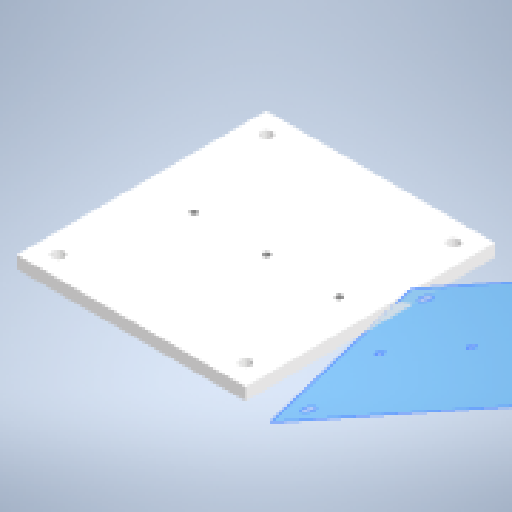
# Autodesk Inventor part: Deska izolovaná
Saved by Autodesk Inventor 2023 (Build 270158000, 158)
## iProperties
Created: 2023-03-26
Part Number: Deska izolovaná
Material: PC/ABS Plastic
Document SubType Name: Modeling
Designer: lukyv
Density: 0.357273 g/cm^3
Appearance: Smooth - White
Author: lukyv
Autodesk Inventor part; units mm, degrees
ref_plane "YZ Plane" through (0, 0, 0) normal (1, 0, 0) x (0, 1, 0)
ref_plane "XZ Plane" through (0, 0, 0) normal (0, 1, 0) x (-1, 0, 0)
ref_plane "XY Plane" through (0, 0, 0) normal (0, 0, 1) x (1, 0, 0)
sketch "Sketch1" plane through (0, 0, 0) normal (0, 1, 0) x (-1, 0, 0)
  line L0 (0, 0) -> (110, 0)
  line L1 (110, 0) -> (110, -110)
  line L2 (110, -110) -> (0, -110)
  line L3 (0, -110) -> (0, 0)
  circle A0 centre (5, -5) radius 2.75
  line L4 (55, 0) -> (55, -110) construction
  line L5 (0, -55) -> (110, -55) construction
  circle A1 centre (5, -105) radius 2.75
  circle A2 centre (105, -5) radius 2.75
  circle A3 centre (105, -105) radius 2.75
  dimension "d0" = 110
  dimension "d1" = 110
  dimension "d2" = 5.5
  dimension "d5" = 100
  dimension "d8" = 100
  dimension "d11" = 5
  dimension "d12" = 5
  constraints: 12 end point, 4 centre point, 4 midpoint, 2 horizontal, 2 parallel, 1 perpendicular, 1 vertical, 6 other
  measures "d0" distance of L1.end L2.end
  measures "d1" distance of L0.end L1.end
  measures "d2" diameter of A0
  measures "d5" distance of A0.centre A1.centre
  measures "d8" distance of A0.centre A2.centre
  measures "d11" distance from line of L0 A0.centre
  measures "d12" distance from line of L3 A0.centre
extrude "Extrusion1" add sketch "Sketch1" along normal blind 6
sketch "Sketch2" plane through (0, 6, 0) normal (0, 1, 0) x (1, 0, 0)
  line L0 (0, 0) -> (0, 110) construction
  line L1 (0, 55) -> (-110, 55) construction
  line L2 (-110, 110) -> (-110, 0) construction
  line L3 (-110, 0) -> (0, 0) construction
  line L4 (-55, 0) -> (-55, 110) construction
  line L5 (0, 110) -> (-110, 110) construction
  circle A0 centre (-20, 55) radius 1.65
  circle A1 centre (-55, 55) radius 1.65
  circle A2 centre (-90, 55) radius 1.65
  point P0 (-110, 7.25)
  point P1 (-2.25, 110)
  dimension "d18" = 3.3
  dimension "d22" = 20
  dimension "d36" = 35
  constraints: 4 end point, 4 midpoint, 3 centre point, 1 horizontal, 1 point on line, 4 other
  measures "d18" diameter of A0
  measures "d22" distance from line of A0.centre L0
  measures "d36" distance of A0.centre A1.centre
extrude "Extrusion2" cut sketch "Sketch2" against normal blind 6
thread "Thread1" size "M4x0.7" class "6H" standard "ANSI Metric M Profile" full length
thread "Thread2" size "M3.5x0.6" class "6H" standard "ANSI Metric M Profile" full length
thread "Thread3" size "M3.5x0.6" class "6H" standard "ANSI Metric M Profile" full length
body "Solid1"
